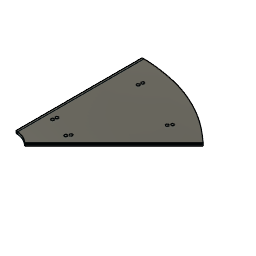
Wheelchair-Spokeguard (Autodesk Fusion 360 design; units mm, degrees)
Autodesk Fusion 360 part; units mm, degrees
note: some values were not read from the file. Set by a fixed rule: which sketch regions a step uses.
sketch "Sketch1" plane through (0, 0, 0) normal (0, 0, 1) x (1, 0, 0)
sketch "Sketch2" plane through (0, 0, 0) normal (0, 0, 1) x (1, 0, 0)
  line L0 (0, 38.1) -> (0, 266.7)
  line L1 (0, 266.7) -> (5.8749, 266.7) construction
  line L2 (5.8749, 266.7) -> (13.1121, 266.7) construction
  line L3 (13.1121, 266.7) -> (25.8544, 265.4439) construction
  line L4 (25.8544, 265.4439) -> (44.0755, 263.0328) construction
  line L5 (44.0755, 263.0328) -> (64.8071, 258.7063) construction
  line L6 (64.8071, 258.7063) -> (77.1006, 255.3123) construction
  line L7 (77.1006, 255.3123) -> (89.3691, 251.2808) construction
  line L8 (89.3691, 251.2808) -> (100.5082, 247.0364) construction
  line L9 (100.5082, 247.0364) -> (118.4009, 238.9772) construction
  line L10 (118.4009, 238.9772) -> (132.3058, 231.5687) construction
  line L11 (132.3058, 231.5687) -> (148.9129, 221.2551) construction
  line L12 (148.9129, 221.2551) -> (168.603, 206.6444) construction
  line L13 (168.603, 206.6444) -> (188.5854, 188.5854) construction
  spline S0 degree 5 poles (0, 266.7) (5.8749, 266.7) (13.1121, 266.7) (25.8544, 265.4439) (44.0755, 263.0328) (64.8071, 258.7063) (77.1006, 255.3123) (89.3691, 251.2808) (100.5082, 247.0364) (118.4009, 238.9772) (132.3058, 231.5687) (148.9129, 221.2551) (168.603, 206.6444) (188.5854, 188.5854) knots 0 0 0 0 0 0 0.111111 0.222222 0.333333 0.444444 0.555556 0.666667 0.777778 0.888889 1 1 1 1 1 1
  line L14 (0, 38.1) -> (3.3782, 38.1) construction
  line L15 (3.3782, 38.1) -> (7.8381, 37.285) construction
  line L16 (7.8381, 37.285) -> (11.1378, 36.4357) construction
  line L17 (11.1378, 36.4357) -> (15.4569, 34.8237) construction
  line L18 (15.4569, 34.8237) -> (19.6708, 32.6292) construction
  line L19 (19.6708, 32.6292) -> (23.4764, 30.0078) construction
  line L20 (23.4764, 30.0078) -> (26.9408, 26.9408) construction
  spline S1 degree 5 poles (0, 38.1) (3.3782, 38.1) (7.8381, 37.285) (11.1378, 36.4357) (15.4569, 34.8237) (19.6708, 32.6292) (23.4764, 30.0078) (26.9408, 26.9408) knots 0 0 0 0 0 0 0.333333 0.666667 1 1 1 1 1 1
  line L21 (26.9408, 26.9408) -> (188.5854, 188.5854)
  constraint vertical L0
extrude "Extrude1" add sketch "Sketch2" along normal blind 4
sketch "Sketch3" plane through (0, 0, 4) normal (0, 0, 1) x (-1, 0, 0)
  spline S0 degree 5 poles (0, -38.1) (-3.3782, -38.1) (-7.8381, -37.285) (-11.1378, -36.4357) (-15.4569, -34.8237) (-19.6708, -32.6292) (-23.4764, -30.0078) (-26.9408, -26.9408) knots 0 0 0 0 0 0 0.333333 0.666667 1 1 1 1 1 1
  line L0 (-26.9408, -26.9408) -> (-188.5854, -188.5854)
  spline S1 degree 5 poles (-188.5854, -188.5854) (-168.603, -206.6444) (-148.9129, -221.2551) (-132.3058, -231.5687) (-118.4009, -238.9772) (-100.5082, -247.0364) (-89.3691, -251.2808) (-77.1006, -255.3123) (-64.8071, -258.7063) (-44.0755, -263.0328) (-25.8544, -265.4439) (-13.1121, -266.7) (-5.8749, -266.7) (0, -266.7) knots -1 -1 -1 -1 -1 -1 -0.888889 -0.777778 -0.666667 -0.555556 -0.444444 -0.333333 -0.222222 -0.111111 0 0 0 0 0 0
  line L1 (0, -266.7) -> (0, -38.1)
  line L2 (0, 0) -> (-46.1934, -262.2689)
  line L3 (0, 0) -> (-152.4933, -218.1326)
  circle A0 centre (-40.1223, -227.7995) radius 2.5
  circle A1 centre (-38.8894, -220.7995) radius 2.5
  circle A2 centre (-132.4397, -189.4472) radius 2.5
  circle A3 centre (-128.429, -183.7101) radius 2.5
  circle A4 centre (-15.6402, -88.7995) radius 2.5
  circle A5 centre (-16.8731, -95.7995) radius 2.5
  circle A6 centre (-56.8091, -81.2621) radius 2.5
  circle A7 centre (-52.7984, -75.525) radius 2.5
  dimension "d5" = 5
  dimension "d6" = 5
  dimension "d7" = 5
  dimension "d8" = 5
  dimension "d9" = 5
  dimension "d10" = 5
  dimension "d11" = 5
  dimension "d12" = 5
  dimension "d13" = 7
  dimension "d14" = 7
  dimension "d15" = 7
  dimension "d16" = 7
  dimension "d17" = 35
  dimension "d18" = 35
  dimension "d19" = 125
  dimension "d20" = 125
  constraint coincident L2.start L3.start
  constraint coincident S1 L2.end
  constraint coincident S1 L3.end
  constraint coincident L2 A0.centre
  constraint coincident L2 A1.centre
  constraint coincident L3 A2.centre
  constraint coincident L3 A3.centre
  constraint coincident L2 A4.centre
  constraint coincident L2 A5.centre
  constraint coincident L3 A6.centre
  constraint coincident L3 A7.centre
  measures "d5" diameter of A2
  measures "d6" diameter of A3
  measures "d7" diameter of A7
  measures "d8" diameter of A6
  measures "d9" diameter of A4
  measures "d10" diameter of A5
  measures "d11" diameter of A1
  measures "d12" diameter of A0
  measures "d13" distance of A2.centre A3.centre
  measures "d14" vertical distance of A0.centre A1.centre
  measures "d15" distance of A6.centre A7.centre
  measures "d16" vertical distance of A4.centre A5.centre
  measures "d17" distance of L3.end A2.centre
  measures "d18" distance of L2.end A0.centre
  measures "d19" distance of A3.centre A6.centre
  measures "d20" vertical distance of A1.centre A5.centre
hole "Hole1" at (15.6402, 88.7995, 4) at (16.8731, 95.7995, 4) at (38.8894, 220.7995, 4) at (40.1223, 227.7995, 4) at (132.4397, 189.4472, 4) at (128.429, 183.7101, 4) at (56.8091, 81.2621, 4) at (52.7984, 75.525, 4) direction (0, 0, -1) diameter 5 depth 5 tip angle 118
sketch "Sketch4" plane through (0, 0, 0) normal (-1, 0, 0) x (0, -1, 0)
  line L0 (-266.7, 0) -> (-38.1, 0)
  line L1 (-38.1, 0) -> (-38.1, 4)
  line L2 (-38.1, 4) -> (-266.7, 4)
  line L3 (-266.7, 4) -> (-266.7, 0)
  line L4 (-38.1, 1.25) -> (-266.7, 1.25)
  line L5 (-266.7, 1.25) -> (-266.7, 2.75)
  line L6 (-266.7, 2.75) -> (-38.1, 2.75)
  line L7 (-38.1, 2.75) -> (-38.1, 1.25)
  dimension "d24" = 1.25
  dimension "d25" = 1.25
  constraint horizontal L4
  constraint vertical L5
  constraint horizontal L6
  constraint vertical L7
  constraint coincident L3 L5.end
  constraint coincident L1 L4.start
  measures "d24" distance of L0 L4
  measures "d25" distance of L2 L6
sketch "Sketch5" plane through (0, 0, 0) normal (0.707107, -0.707107, 0) x (0.707107, 0.707107, 0)
  line L0 (38.1, 0) -> (266.7, 0)
  line L1 (266.7, 0) -> (266.7, 4)
  line L2 (266.7, 4) -> (38.1, 4)
  line L3 (38.1, 4) -> (38.1, 0)
  line L4 (266.7, 1.25) -> (38.1, 1.25)
  line L5 (38.1, 1.25) -> (38.1, 2.75)
  line L6 (38.1, 2.75) -> (266.7, 2.75)
  line L7 (266.7, 2.75) -> (266.7, 1.25)
  dimension "d26" = 1.25
  dimension "d27" = 1.25
  constraint horizontal L4
  constraint vertical L5
  constraint horizontal L6
  constraint vertical L7
  constraint coincident L3 L5.end
  constraint coincident L1 L4.start
  measures "d26" distance of L0 L4
  measures "d27" distance of L2 L6
extrude "Extrude2" add sketch "Sketch5" along normal blind 3 contours L1 L3 L4 L5 L6 L7
extrude "Extrude3" cut sketch "Sketch4" against normal blind 3 contours L1 L3 L4 L5 L6 L7
sketch "Sketch6" plane through (26.9408, 26.9408, 0) normal (-0.707107, -0.707107, 0) x (0.707107, -0.707107, 0)
  line L0 (0, 2.75) -> (0, 1.25)
  line L1 (0, 1.25) -> (3, 1.25)
  line L2 (3, 1.25) -> (3, 2.75)
  line L3 (3, 2.75) -> (0, 2.75)
  line L4 (3, 1.25) -> (3, 0.75)
  line L5 (3, 3.25) -> (4.0534, 3.25)
  line L6 (4.0534, 0.75) -> (3, 0.75)
  line L7 (3, 0.75) -> (3, 3.25)
  line L8 (3, 3.25) -> (3, 0.75)
  line L9 (0, 1.25) -> (3, 0.75)
  line L10 (3, 3.25) -> (0, 2.75)
  dimension "d32" = 0.5
  dimension "d33" = 0.5
  dimension "d34" = 2.5
  constraint coincident L1.end L2.start
  constraint perpendicular L1 L4
  constraint horizontal L5
  constraint horizontal L6
  constraint vertical L7
  constraint perpendicular L6 L8
  constraint coincident L0.end L1.start
  constraint coincident L0.start L3.end
  measures "d32" distance of L2.end L5.start
  measures "d33" distance of L1.end L4.end
  measures "d34" distance of L5.end L6.start
extrude "Extrude4" add sketch "Sketch6" against normal blind 228.6 contours L3 L7 L8 L10 | L1 L4 L7 L8 L9
sketch "Sketch7" plane through (0, 0, 0) normal (0, 0, -1) x (1, 0, 0)
  circle A0 centre (56.8091, -81.2621) radius 2.5
  circle A1 centre (132.4397, -189.4472) radius 2.5
  circle A2 centre (38.8894, -220.7995) radius 2.5
  circle A3 centre (15.6402, -88.7995) radius 2.5
  circle A4 centre (16.8731, -95.7995) radius 2.5
  circle A5 centre (40.1223, -227.7995) radius 2.5
  circle A6 centre (128.429, -183.7101) radius 2.5
  circle A7 centre (52.7984, -75.525) radius 2.5
  spline S0 degree 5 poles (0, -38.1) (3.3782, -38.1) (7.8381, -37.285) (11.1378, -36.4357) (15.4569, -34.8237) (19.6708, -32.6292) (23.4764, -30.0078) (26.9408, -26.9408) knots 0 0 0 0 0 0 0.333333 0.666667 1 1 1 1 1 1
  line L0 (0, -38.1) -> (0, -266.7)
  spline S1 degree 5 poles (0, -266.7) (5.8749, -266.7) (13.1121, -266.7) (25.8544, -265.4439) (44.0755, -263.0328) (64.8071, -258.7063) (77.1006, -255.3123) (89.3691, -251.2808) (100.5082, -247.0364) (118.4009, -238.9772) (132.3058, -231.5687) (148.9129, -221.2551) (168.603, -206.6444) (188.5854, -188.5854) knots 0 0 0 0 0 0 0.111111 0.222222 0.333333 0.444444 0.555556 0.666667 0.777778 0.888889 1 1 1 1 1 1
  line L1 (188.5854, -188.5854) -> (26.9408, -26.9408)
sketch "Sketch8" plane through (0, 0, 0) normal (1, 0, 0) x (0, 1, 0)
sketch "Sketch9" plane through (0, 0, 2.75) normal (0, 0, -1) x (1, 0, 0)
  spline S0 degree 3 poles (3, -266.6974) (2.0462, -266.7) (1.0538, -266.7) (0, -266.7) knots -0.31615 -0.31615 -0.31615 -0.31615 0 0 0 0
  line L0 (3, -266.6974) -> (3, -38.1)
  line L1 (3, -38.1) -> (0, -38.1)
  line L2 (0, -38.1) -> (0, -266.7)
sketch "Sketch10" plane through (0, 0, 0) normal (0, 0, -1) x (1, 0, 0)
sketch "Sketch11" plane through (0, 0, 0) normal (0, 1, 0) x (1, 0, 0)
  line L0 (0, -2.75) -> (0, -1.25)
  line L1 (3, -2.75) -> (3, -3.25)
  line L2 (3, -3.25) -> (3, -0.75)
  line L3 (0, -2.75) -> (3, -3.25)
  line L4 (0, -1.25) -> (3, -0.75)
  dimension "d44" = 1.5
  dimension "d47" = 0.5
  dimension "d48" = 2.5
  measures "d44" distance of L0.end L0.start
  measures "d47" distance of L1.start L1.end
  measures "d48" distance of L1.end L2.end
extrude "Extrude5" cut sketch "Sketch11" along normal blind 309
